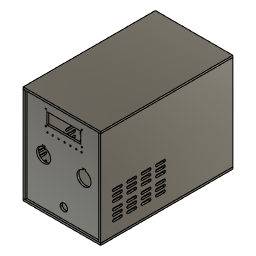
lazy-welder-chassis (Autodesk Fusion 360 design; units mm, degrees)
Autodesk Fusion 360 part; units mm, degrees
sketch "Sketch1" plane through (0, 0, 0) normal (0, 1, 0) x (1, 0, 0)
  line L0 (0, 0) -> (0, -197.9)
  line L1 (0, -197.9) -> (153.8, -197.9)
  line L2 (153.8, -197.9) -> (153.8, 0)
  line L3 (153.8, 0) -> (0, 0)
  line L4 (41.45, -177.9) -> (112.35, -177.9)
  line L5 (112.35, -177.9) -> (112.35, -153.9)
  line L6 (112.35, -153.9) -> (41.45, -153.9)
  line L7 (41.45, -153.9) -> (41.45, -177.9)
  circle A0 centre (39.4, -181.4) radius 1.5
  circle A1 centre (102.95, -140.7) radius 1.5
  circle A2 centre (113.95, -140.7) radius 1.5
  circle A3 centre (90.65, -140.7) radius 1.5
  circle A4 centre (78.35, -140.7) radius 1.5
  circle A5 centre (66.05, -140.7) radius 1.5
  circle A6 centre (53.75, -140.7) radius 1.5
  circle A7 centre (42.75, -140.7) radius 1.5
  circle A8 centre (114.4, -181.4) radius 1.5
  line L8 (31.8, -113.1111) -> (37.6, -113.1111)
  line L9 (31.8, -113.1111) -> (31.8, -110.1111)
  line L10 (37.6, -113.1111) -> (37.6, -110.1111)
  arc A9 (37.6, -110.1111) -> (31.8, -110.1111) centre (34.7, -95.7) ccw
  line L11 (116.2, -113.1111) -> (122, -113.1111)
  line L12 (116.2, -113.1111) -> (116.2, -110.1111)
  line L13 (122, -113.1111) -> (122, -110.1111)
  arc A10 (122, -110.1111) -> (116.2, -110.1111) centre (119.1, -95.7) ccw
  circle A11 centre (114.4, -150.4) radius 1.5
  circle A12 centre (39.4, -150.4) radius 1.5
  line L14 (69.55, -25.0076) -> (69.55, -20.0924)
  line L15 (84.25, -25.0076) -> (84.25, -20.0924)
  arc A13 (69.55, -25.0076) -> (84.25, -25.0076) centre (76.9, -22.55) ccw
  arc A14 (84.25, -20.0924) -> (69.55, -20.0924) centre (76.9, -22.55) ccw
  point P0 (106.0012, -102.3717)
  point P1 (41.7115, -182.3254)
  dimension "d1" = 197.9
  dimension "d6" = 70.9
  dimension "d13" = 153.8
  dimension "d22" = 29.4
  dimension "d27" = 95.7
  dimension "d28" = 34.7
  dimension "d29" = 84.4
  dimension "d30" = 95.7
  dimension "d31" = 34.7
  dimension "d32" = 22.55
  dimension "d33" = 76.9
  dimension "d34" = 20
  dimension "d35" = 41.45
  dimension "d38" = 3
  dimension "d39" = 13.2
  dimension "d40" = 9.4
  dimension "d41" = 3
  dimension "d42" = 11
  dimension "d43" = 13.2
  dimension "d44" = 3
  dimension "d45" = 3
  dimension "d46" = 12.3
  dimension "d47" = 12.3
  dimension "d49" = 12.3
  dimension "d50" = 3
  dimension "d51" = 12.3
  dimension "d52" = 3
  dimension "d53" = 11
  dimension "d54" = 13.2
  dimension "d55" = 13.2
  dimension "d56" = 13.2
  dimension "d57" = 13.2
  dimension "d58" = 3
  dimension "d59" = 13.2
  dimension "d60" = 3
  dimension "d61" = 75
  dimension "d69" = 5.8
  dimension "d70" = 3
  dimension "d71" = 3
  dimension "d72" = 5.8
  dimension "d73" = 3
  dimension "d74" = 3
  dimension "d77" = 3
  dimension "d78" = 3
  dimension "d80" = 31
  dimension "d81" = 31
  dimension "d82" = 24
  dimension "d83" = 3.5
  dimension "d86" = 75
  dimension "d87" = 2.05
  dimension "d89" = 3
  dimension "d94" = 14.7
  dimension "d101" = 14.7
  dimension "d102" = 7.75
  constraint coincident L0.start L3.end
  constraint vertical L0
  constraint perpendicular L0 L1
  constraint perpendicular L1 L2
  constraint perpendicular L0 L3
  constraint horizontal L4
  constraint vertical L5
  constraint horizontal L6
  constraint vertical L7
  constraint coincident P0 A10
  constraint horizontal L8
  constraint perpendicular L8 L9
  constraint perpendicular L8 L10
  constraint horizontal L11
  constraint perpendicular L11 L12
  constraint perpendicular L11 L13
  constraint vertical L14
  constraint coincident L15.end A13
  constraint vertical L15
  constraint concentric A13 A14
  measures "d1" distance of L0.start L0.end
  measures "d6" distance of L4.start L4.end
  measures "d13" distance of L0.end L1.end
  measures "d22" diameter of A9
  measures "d27" distance of L3 A9.centre
  measures "d28" distance of L0 A9.centre
  measures "d29" horizontal distance of A10.centre A9.centre
  measures "d30" distance of L3 A10.centre
  measures "d31" distance of L2 A10.centre
  measures "d32" distance of L3 A13.centre
  measures "d33" distance of L0 A13.centre
  measures "d34" distance of L1 L4
  measures "d35" distance of L0 L7
  measures "d38" diameter of A1
  measures "d39" distance of L6 A1.centre
  measures "d40" distance of L5 A1.centre
  measures "d41" diameter of A2
  measures "d42" horizontal distance of A1.centre A2.centre
  measures "d43" distance of L6 A2.centre
  measures "d44" diameter of A3
  measures "d45" diameter of A4
  measures "d46" horizontal distance of A1.centre A3.centre
  measures "d47" horizontal distance of A3.centre A4.centre
  measures "d49" horizontal distance of A4.centre A5.centre
  measures "d50" diameter of A6
  measures "d51" horizontal distance of A5.centre A6.centre
  measures "d52" diameter of A7
  measures "d53" distance of A6.centre A7.centre
  measures "d54" distance of L6 A3.centre
  measures "d55" distance of L6 A4.centre
  measures "d56" distance of L6 A5.centre
  measures "d57" distance of L6 A6.centre
  measures "d58" diameter of A5
  measures "d59" distance of L6 A7.centre
  measures "d60" diameter of A8
  measures "d61" horizontal distance of A0.centre A8.centre
  measures "d69" distance of L8.start L8.end
  measures "d70" distance of L8.start L9.end
  measures "d71" distance of L8.end L10.end
  measures "d72" distance of L11.start L11.end
  measures "d73" distance of L11.start L12.end
  measures "d74" distance of L11.end L13.end
  measures "d77" diameter of A11
  measures "d78" diameter of A12
  measures "d80" vertical distance of A8.centre A11.centre
  measures "d81" vertical distance of A0.centre A12.centre
  measures "d82" distance of L4.start L6.end
  measures "d83" distance of L4 A0.centre
  measures "d86" distance of A11.centre A12.centre
  measures "d87" distance of L7 A0.centre
  measures "d89" diameter of A0
  measures "d94" radius of A10
  measures "d101" distance of L14 L15
  measures "d102" radius of A13
sketch "Sketch3" plane through (0, 0, 0) normal (0, 1, 0) x (1, 0, 0)
  line L0 (0, -197.9) -> (153.8, -197.9)
  line L1 (153.8, -197.9) -> (153.8, 0)
  line L2 (153.8, 0) -> (0, 0)
  circle A0 centre (99.4, -30) radius 1.7
  circle A1 centre (139.4, -30) radius 1.7
  line L3 (112.4711, -40) -> (126.3289, -40)
  line L4 (133.4, -32.9289) -> (133.4, -24)
  line L5 (129.4, -20) -> (109.4, -20)
  line L6 (105.4, -24) -> (105.4, -32.9289)
  line L7 (105.4, -32.9289) -> (112.4711, -40)
  line L8 (105.4, -32.9289) -> (47.9841, -32.9289) construction
  line L9 (126.3289, -40) -> (133.4, -32.9289)
  line L10 (126.3289, -40) -> (50.3873, -40) construction
  arc A2 (133.4, -24) -> (129.4, -20) centre (129.4, -24) ccw
  arc A3 (109.4, -20) -> (105.4, -24) centre (109.4, -24) ccw
  line L11 (105, -71.5) -> (133.8, -71.5)
  line L12 (133.8, -71.5) -> (133.8, -50)
  line L13 (133.8, -50) -> (105, -50)
  line L14 (105, -50) -> (105, -71.5)
  circle A4 centre (22.5, -175.4037) radius 2.15
  circle A5 centre (22.5, -143.4037) radius 2.15
  circle A6 centre (54.5073, -143.4037) radius 2.15
  circle A7 centre (54.5, -175.4037) radius 2.15
  circle A8 centre (99.3, -175.4037) radius 2.15
  circle A9 centre (99.3, -143.4037) radius 2.15
  circle A10 centre (131.3, -175.4037) radius 2.15
  circle A11 centre (131.3, -143.4037) radius 2.15
  circle A12 centre (38.5, -159.4) radius 18.5
  circle A13 centre (115.3, -159.4) radius 18.5
  line L15 (0, -20) -> (17.5, -20)
  line L16 (17.5, -20) -> (17.5, -100)
  line L17 (17.5, -100) -> (0, -100)
  line L18 (0, 0) -> (0, -20)
  line L19 (0, -100) -> (0, -197.9)
  dimension "d103" = 197.9
  dimension "d104" = 153.8
  dimension "d105" = 3.4
  dimension "d106" = 3.4
  dimension "d109" = 4
  dimension "d110" = 4
  dimension "d117" = 10
  dimension "d121" = 10
  dimension "d124" = 6
  dimension "d125" = 6
  dimension "d126" = 40
  dimension "d127" = 10
  dimension "d128" = 10
  dimension "d129" = 28.8
  dimension "d130" = 21.5
  dimension "d131" = 20
  dimension "d133" = 20
  dimension "d134" = 20
  dimension "d135" = 50
  dimension "d136" = 4.3
  dimension "d137" = 4.3
  dimension "d138" = 4.3
  dimension "d139" = 4.3
  dimension "d140" = 4.3
  dimension "d141" = 4.3
  dimension "d142" = 4.3
  dimension "d143" = 4.3
  dimension "d144" = 32
  dimension "d145" = 32
  dimension "d148" = 32
  dimension "d149" = 32
  dimension "d150" = 32
  dimension "d151" = 37
  dimension "d152" = 22.63
  dimension "d153" = 22.63
  dimension "d154" = 22.63
  dimension "d155" = 22.6248
  dimension "d156" = 38.5
  dimension "d157" = 38.5
  dimension "d158" = 32
  dimension "d159" = 32
  dimension "d160" = 32
  dimension "d161" = 32
  dimension "d162" = 32
  dimension "d163" = 32
  dimension "d164" = 37
  dimension "d165" = 22.63
  dimension "d166" = 22.63
  dimension "d167" = 22.6248
  dimension "d168" = 22.6248
  dimension "d169" = 38.5
  dimension "d170" = 38.5
  dimension "d310" = 20.4
  dimension "d311" = 17.5
  dimension "d312" = 80
  dimension "d313" = 20
  constraint coincident L2.end L18.start
  constraint vertical L18
  constraint perpendicular L0 L18
  constraint perpendicular L0 L1
  constraint perpendicular L2 L18
  constraint horizontal L3
  constraint vertical L4
  constraint horizontal L5
  constraint vertical L6
  constraint tangent L6 A3
  constraint tangent L5 A3
  constraint tangent L4 A2
  constraint tangent L5 A2
  constraint horizontal L8
  constraint horizontal L10
  constraint horizontal L11
  constraint vertical L12
  constraint horizontal L13
  constraint vertical L14
  constraint perpendicular L15 L18
  constraint perpendicular L15 L16
  constraint coincident L17.end L18
  constraint perpendicular L17 L18
  constraint collinear L18 L19
  measures "d103" distance of L2.end L0.start
  measures "d104" distance of L0.start L0.end
  measures "d105" diameter of A0
  measures "d106" diameter of A1
  measures "d109" radius of A3
  measures "d110" radius of A2
  measures "d117" distance of A0.centre L3
  measures "d121" distance of A1.centre L3
  measures "d124" distance of A0.centre L6
  measures "d125" distance of A1.centre L4
  measures "d126" distance of A0.centre A1.centre
  measures "d127" distance of L6.end L3.start
  measures "d128" distance of L3.end L4.start
  measures "d129" distance of L11.start L11.end
  measures "d130" distance of L11.start L13.end
  measures "d131" distance of L3 L5
  measures "d133" distance of L2 L5
  measures "d134" distance of L1 L12
  measures "d135" distance of L2 L13
  measures "d136" diameter of A4
  measures "d137" diameter of A5
  measures "d138" diameter of A6
  measures "d139" diameter of A7
  measures "d140" diameter of A8
  measures "d141" diameter of A9
  measures "d142" diameter of A10
  measures "d143" diameter of A11
  measures "d144" horizontal distance of A4.centre A7.centre
  measures "d145" vertical distance of A4.centre A5.centre
  measures "d148" vertical distance of A5.centre A7.centre
  measures "d149" horizontal distance of A5.centre A7.centre
  measures "d150" distance of A6.centre A7.centre
  measures "d151" diameter of A12
  measures "d152" distance of A4.centre A12.centre
  measures "d153" distance of A7.centre A12.centre
  measures "d154" distance of A6.centre A12.centre
  measures "d155" distance of A5.centre A12.centre
  measures "d156" distance of L0 A12.centre
  measures "d157" distance of A12.centre L18
  measures "d158" horizontal distance of A8.centre A10.centre
  measures "d159" horizontal distance of A9.centre A10.centre
  measures "d160" horizontal distance of A8.centre A11.centre
  measures "d161" distance of A8.centre A9.centre
  measures "d162" vertical distance of A8.centre A11.centre
  measures "d163" distance of A10.centre A11.centre
  measures "d164" diameter of A13
  measures "d165" distance of A8.centre A13.centre
  measures "d166" distance of A10.centre A13.centre
  measures "d167" distance of A9.centre A13.centre
  measures "d168" distance of A11.centre A13.centre
  measures "d169" distance of L0 A13.centre
  measures "d170" distance of L1 A13.centre
  measures "d310" distance of L1 L4
  measures "d311" distance of L15.start L15.end
  measures "d312" distance of L15.end L16.end
  measures "d313" distance of L2 L15
extrude "Extrude3" add sketch "Sketch1" along normal blind 4 makes body 1
extrude "Extrude4" add sketch "Sketch3" along normal blind 4 separate body makes body 2
move_face "MoveFace1" by (0, 0, 260) 1 faces at (153.8, 1.3333, 131.9333) on bodies 2
move_body "Move1" bodies 2 to x (1, 0, 0) y (0, 1, 0) z (0, 0, 1) at (0, 263, 0)
sketch "Sketch4" plane through (0, 0, 0) normal (1, 0, 0) x (0, 1, 0)
  line L0 (0, 0) -> (0, 197.9)
  line L1 (0, 197.9) -> (276, 197.9)
  line L2 (276, 197.9) -> (276, 0)
  line L3 (276, 0) -> (0, 0)
  line L4 (27, 30) -> (43, 30)
  line L5 (45, 28) -> (45, 27)
  line L6 (43, 25) -> (27, 25)
  line L7 (25, 27) -> (25, 28)
  arc A0 (27, 30) -> (25, 28) centre (27, 28) ccw
  arc A1 (25, 27) -> (27, 25) centre (27, 27) ccw
  arc A2 (45, 28) -> (43, 30) centre (43, 28) ccw
  arc A3 (43, 25) -> (45, 27) centre (43, 27) ccw
  arc A4 (45, 38) -> (43, 40) centre (43, 38) ccw
  line L8 (43, 35) -> (27, 35)
  arc A5 (43, 35) -> (45, 37) centre (43, 37) ccw
  line L9 (27, 40) -> (43, 40)
  line L10 (45, 38) -> (45, 37)
  arc A6 (27, 40) -> (25, 38) centre (27, 38) ccw
  arc A7 (25, 37) -> (27, 35) centre (27, 37) ccw
  line L11 (25, 37) -> (25, 38)
  arc A8 (45, 48) -> (43, 50) centre (43, 48) ccw
  line L12 (43, 45) -> (27, 45)
  arc A9 (43, 45) -> (45, 47) centre (43, 47) ccw
  line L13 (27, 50) -> (43, 50)
  line L14 (45, 48) -> (45, 47)
  arc A10 (27, 50) -> (25, 48) centre (27, 48) ccw
  arc A11 (25, 47) -> (27, 45) centre (27, 47) ccw
  line L15 (25, 47) -> (25, 48)
  arc A12 (75, 28) -> (73, 30) centre (73, 28) ccw
  line L16 (73, 25) -> (57, 25)
  arc A13 (73, 25) -> (75, 27) centre (73, 27) ccw
  line L17 (57, 30) -> (73, 30)
  line L18 (75, 28) -> (75, 27)
  arc A14 (57, 30) -> (55, 28) centre (57, 28) ccw
  arc A15 (55, 27) -> (57, 25) centre (57, 27) ccw
  line L19 (55, 27) -> (55, 28)
  arc A16 (75, 38) -> (73, 40) centre (73, 38) ccw
  line L20 (73, 35) -> (57, 35)
  arc A17 (73, 35) -> (75, 37) centre (73, 37) ccw
  line L21 (57, 40) -> (73, 40)
  line L22 (75, 38) -> (75, 37)
  arc A18 (57, 40) -> (55, 38) centre (57, 38) ccw
  arc A19 (55, 37) -> (57, 35) centre (57, 37) ccw
  line L23 (55, 37) -> (55, 38)
  arc A20 (75, 48) -> (73, 50) centre (73, 48) ccw
  line L24 (73, 45) -> (57, 45)
  arc A21 (73, 45) -> (75, 47) centre (73, 47) ccw
  line L25 (57, 50) -> (73, 50)
  line L26 (75, 48) -> (75, 47)
  arc A22 (57, 50) -> (55, 48) centre (57, 48) ccw
  arc A23 (55, 47) -> (57, 45) centre (57, 47) ccw
  line L27 (55, 47) -> (55, 48)
  arc A24 (105, 28) -> (103, 30) centre (103, 28) ccw
  line L28 (103, 25) -> (87, 25)
  arc A25 (103, 25) -> (105, 27) centre (103, 27) ccw
  line L29 (87, 30) -> (103, 30)
  line L30 (105, 28) -> (105, 27)
  arc A26 (87, 30) -> (85, 28) centre (87, 28) ccw
  arc A27 (85, 27) -> (87, 25) centre (87, 27) ccw
  line L31 (85, 27) -> (85, 28)
  arc A28 (105, 38) -> (103, 40) centre (103, 38) ccw
  line L32 (103, 35) -> (87, 35)
  arc A29 (103, 35) -> (105, 37) centre (103, 37) ccw
  line L33 (87, 40) -> (103, 40)
  line L34 (105, 38) -> (105, 37)
  arc A30 (87, 40) -> (85, 38) centre (87, 38) ccw
  arc A31 (85, 37) -> (87, 35) centre (87, 37) ccw
  line L35 (85, 37) -> (85, 38)
  arc A32 (105, 48) -> (103, 50) centre (103, 48) ccw
  line L36 (103, 45) -> (87, 45)
  arc A33 (103, 45) -> (105, 47) centre (103, 47) ccw
  line L37 (87, 50) -> (103, 50)
  line L38 (105, 48) -> (105, 47)
  arc A34 (87, 50) -> (85, 48) centre (87, 48) ccw
  arc A35 (85, 47) -> (87, 45) centre (87, 47) ccw
  line L39 (85, 47) -> (85, 48)
  arc A36 (135, 28) -> (133, 30) centre (133, 28) ccw
  line L40 (133, 25) -> (117, 25)
  arc A37 (133, 25) -> (135, 27) centre (133, 27) ccw
  line L41 (117, 30) -> (133, 30)
  line L42 (135, 28) -> (135, 27)
  arc A38 (117, 30) -> (115, 28) centre (117, 28) ccw
  arc A39 (115, 27) -> (117, 25) centre (117, 27) ccw
  line L43 (115, 27) -> (115, 28)
  arc A40 (135, 38) -> (133, 40) centre (133, 38) ccw
  line L44 (133, 35) -> (117, 35)
  arc A41 (133, 35) -> (135, 37) centre (133, 37) ccw
  line L45 (117, 40) -> (133, 40)
  line L46 (135, 38) -> (135, 37)
  arc A42 (117, 40) -> (115, 38) centre (117, 38) ccw
  arc A43 (115, 37) -> (117, 35) centre (117, 37) ccw
  line L47 (115, 37) -> (115, 38)
  arc A44 (135, 48) -> (133, 50) centre (133, 48) ccw
  line L48 (133, 45) -> (117, 45)
  arc A45 (133, 45) -> (135, 47) centre (133, 47) ccw
  line L49 (117, 50) -> (133, 50)
  line L50 (135, 48) -> (135, 47)
  arc A46 (117, 50) -> (115, 48) centre (117, 48) ccw
  arc A47 (115, 47) -> (117, 45) centre (117, 47) ccw
  line L51 (115, 47) -> (115, 48)
  arc A48 (45, 28) -> (43, 30) centre (43, 28) ccw
  line L52 (43, 25) -> (27, 25)
  arc A49 (43, 25) -> (45, 27) centre (43, 27) ccw
  line L53 (27, 30) -> (43, 30)
  line L54 (45, 28) -> (45, 27)
  arc A50 (27, 30) -> (25, 28) centre (27, 28) ccw
  arc A51 (25, 27) -> (27, 25) centre (27, 27) ccw
  line L55 (25, 27) -> (25, 28)
  line L56 (57, 65) -> (73, 65)
  arc A52 (85, 72) -> (87, 70) centre (87, 72) ccw
  line L57 (85, 62) -> (85, 63)
  arc A53 (73, 70) -> (75, 72) centre (73, 72) ccw
  arc A54 (133, 70) -> (135, 72) centre (133, 72) ccw
  arc A55 (87, 65) -> (85, 63) centre (87, 63) ccw
  arc A56 (115, 72) -> (117, 70) centre (117, 72) ccw
  line L58 (133, 70) -> (117, 70)
  line L59 (55, 82) -> (55, 83)
  arc A57 (105, 73) -> (103, 75) centre (103, 73) ccw
  line L60 (105, 63) -> (105, 62)
  line L61 (75, 83) -> (75, 82)
  arc A58 (55, 72) -> (57, 70) centre (57, 72) ccw
  line L62 (45, 73) -> (45, 72)
  arc A59 (43, 80) -> (45, 82) centre (43, 82) ccw
  arc A60 (85, 62) -> (87, 60) centre (87, 62) ccw
  line L63 (103, 70) -> (87, 70)
  line L64 (45, 63) -> (45, 62)
  line L65 (85, 82) -> (85, 83)
  arc A61 (75, 73) -> (73, 75) centre (73, 73) ccw
  line L66 (45, 63) -> (45, 62)
  line L67 (57, 85) -> (73, 85)
  arc A62 (87, 85) -> (85, 83) centre (87, 83) ccw
  line L68 (73, 60) -> (57, 60)
  line L69 (105, 73) -> (105, 72)
  line L70 (57, 75) -> (73, 75)
  arc A63 (43, 70) -> (45, 72) centre (43, 72) ccw
  line L71 (135, 83) -> (135, 82)
  arc A64 (45, 73) -> (43, 75) centre (43, 73) ccw
  arc A65 (133, 60) -> (135, 62) centre (133, 62) ccw
  arc A66 (55, 82) -> (57, 80) centre (57, 82) ccw
  arc A67 (105, 63) -> (103, 65) centre (103, 63) ccw
  arc A68 (55, 62) -> (57, 60) centre (57, 62) ccw
  line L72 (105, 83) -> (105, 82)
  line L73 (87, 85) -> (103, 85)
  arc A69 (105, 83) -> (103, 85) centre (103, 83) ccw
  line L74 (103, 80) -> (87, 80)
  arc A70 (85, 82) -> (87, 80) centre (87, 82) ccw
  line L75 (43, 60) -> (27, 60)
  line L76 (27, 65) -> (43, 65)
  arc A71 (25, 62) -> (27, 60) centre (27, 62) ccw
  arc A72 (27, 75) -> (25, 73) centre (27, 73) ccw
  line L77 (73, 70) -> (57, 70)
  line L78 (73, 80) -> (57, 80)
  arc A73 (45, 63) -> (43, 65) centre (43, 63) ccw
  arc A74 (45, 83) -> (43, 85) centre (43, 83) ccw
  line L79 (55, 62) -> (55, 63)
  arc A75 (43, 60) -> (45, 62) centre (43, 62) ccw
  line L80 (117, 85) -> (133, 85)
  line L81 (115, 72) -> (115, 73)
  line L82 (135, 73) -> (135, 72)
  line L83 (87, 75) -> (103, 75)
  arc A76 (57, 75) -> (55, 73) centre (57, 73) ccw
  line L84 (85, 72) -> (85, 73)
  arc A77 (103, 70) -> (105, 72) centre (103, 72) ccw
  arc A78 (135, 63) -> (133, 65) centre (133, 63) ccw
  arc A79 (73, 60) -> (75, 62) centre (73, 62) ccw
  arc A80 (43, 60) -> (45, 62) centre (43, 62) ccw
  arc A81 (57, 65) -> (55, 63) centre (57, 63) ccw
  line L85 (75, 73) -> (75, 72)
  arc A82 (87, 75) -> (85, 73) centre (87, 73) ccw
  arc A83 (103, 60) -> (105, 62) centre (103, 62) ccw
  line L86 (55, 72) -> (55, 73)
  line L87 (87, 65) -> (103, 65)
  arc A84 (135, 73) -> (133, 75) centre (133, 73) ccw
  line L88 (117, 65) -> (133, 65)
  arc A85 (45, 63) -> (43, 65) centre (43, 63) ccw
  arc A86 (75, 63) -> (73, 65) centre (73, 63) ccw
  arc A87 (115, 82) -> (117, 80) centre (117, 82) ccw
  arc A88 (75, 83) -> (73, 85) centre (73, 83) ccw
  arc A89 (133, 80) -> (135, 82) centre (133, 82) ccw
  arc A90 (57, 85) -> (55, 83) centre (57, 83) ccw
  line L89 (27, 85) -> (43, 85)
  line L90 (25, 62) -> (25, 63)
  line L91 (27, 75) -> (43, 75)
  line L92 (117, 75) -> (133, 75)
  line L93 (25, 82) -> (25, 83)
  arc A91 (115, 62) -> (117, 60) centre (117, 62) ccw
  line L94 (43, 60) -> (27, 60)
  arc A92 (25, 82) -> (27, 80) centre (27, 82) ccw
  arc A93 (117, 65) -> (115, 63) centre (117, 63) ccw
  line L95 (45, 83) -> (45, 82)
  arc A94 (73, 80) -> (75, 82) centre (73, 82) ccw
  arc A95 (25, 72) -> (27, 70) centre (27, 72) ccw
  line L96 (43, 80) -> (27, 80)
  arc A96 (25, 62) -> (27, 60) centre (27, 62) ccw
  line L97 (115, 82) -> (115, 83)
  line L98 (43, 70) -> (27, 70)
  arc A97 (117, 75) -> (115, 73) centre (117, 73) ccw
  line L99 (135, 63) -> (135, 62)
  arc A98 (117, 85) -> (115, 83) centre (117, 83) ccw
  line L100 (103, 60) -> (87, 60)
  arc A99 (103, 80) -> (105, 82) centre (103, 82) ccw
  arc A100 (27, 65) -> (25, 63) centre (27, 63) ccw
  arc A101 (27, 65) -> (25, 63) centre (27, 63) ccw
  line L101 (27, 65) -> (43, 65)
  line L102 (25, 62) -> (25, 63)
  line L103 (133, 60) -> (117, 60)
  line L104 (133, 80) -> (117, 80)
  line L105 (115, 62) -> (115, 63)
  arc A102 (135, 83) -> (133, 85) centre (133, 83) ccw
  line L106 (25, 72) -> (25, 73)
  line L107 (75, 63) -> (75, 62)
  arc A103 (27, 85) -> (25, 83) centre (27, 83) ccw
  dimension "d178" = 197.9
  dimension "d179" = 276
  dimension "d190" = 2
  dimension "d191" = 2
  dimension "d192" = 2
  dimension "d193" = 2
  dimension "d194" = 2
  dimension "d195" = 2
  dimension "d196" = 2
  dimension "d197" = 2
  dimension "d198" = 2
  dimension "d199" = 2
  dimension "d200" = 2
  dimension "d201" = 2
  dimension "d202" = 2
  dimension "d203" = 2
  dimension "d204" = 2
  dimension "d205" = 2
  dimension "d206" = 2
  dimension "d207" = 2
  dimension "d208" = 2
  dimension "d209" = 2
  dimension "d210" = 2
  dimension "d211" = 2
  dimension "d212" = 2
  dimension "d213" = 2
  dimension "d214" = 2
  dimension "d215" = 2
  dimension "d216" = 2
  dimension "d217" = 2
  dimension "d218" = 2
  dimension "d219" = 2
  dimension "d220" = 2
  dimension "d221" = 2
  dimension "d222" = 2
  dimension "d223" = 2
  dimension "d224" = 2
  dimension "d225" = 2
  dimension "d226" = 2
  dimension "d227" = 2
  dimension "d228" = 2
  dimension "d229" = 2
  dimension "d230" = 2
  dimension "d231" = 2
  dimension "d232" = 2
  dimension "d233" = 2
  dimension "d234" = 2
  dimension "d235" = 2
  dimension "d236" = 2
  dimension "d237" = 2
  dimension "d238" = 2
  dimension "d239" = 2
  dimension "d240" = 2
  dimension "d241" = 2
  dimension "d242" = 2
  dimension "d243" = 2
  dimension "d244" = 2
  dimension "d245" = 2
  dimension "d246" = 2
  dimension "d247" = 2
  dimension "d248" = 2
  dimension "d249" = 2
  dimension "d250" = 2
  dimension "d251" = 2
  dimension "d252" = 2
  dimension "d253" = 2
  dimension "d254" = 2
  dimension "d255" = 2
  dimension "d256" = 2
  dimension "d257" = 2
  dimension "d258" = 2
  dimension "d259" = 2
  dimension "d260" = 2
  dimension "d261" = 2
  dimension "d262" = 2
  dimension "d263" = 2
  dimension "d264" = 2
  dimension "d265" = 2
  dimension "d266" = 2
  dimension "d267" = 2
  dimension "d268" = 2
  dimension "d269" = 2
  dimension "d270" = 2
  dimension "d271" = 2
  dimension "d272" = 2
  dimension "d273" = 2
  dimension "d274" = 2
  dimension "d275" = 2
  dimension "d276" = 2
  dimension "d277" = 2
  dimension "d278" = 2
  dimension "d279" = 2
  dimension "d280" = 2
  dimension "d281" = 2
  dimension "d282" = 2
  dimension "d283" = 2
  dimension "d284" = 2
  dimension "d285" = 2
  dimension "d286" = 2
  dimension "d287" = 2
  dimension "d288" = 2
  dimension "d289" = 2
  dimension "d290" = 2
  dimension "d291" = 2
  dimension "d292" = 2
  dimension "d293" = 2
  constraint coincident L0.start L3.end
  constraint vertical L0
  constraint perpendicular L0 L1
  constraint perpendicular L1 L2
  constraint perpendicular L0 L3
  constraint horizontal L4
  constraint vertical L5
  constraint horizontal L6
  constraint vertical L7
  constraint tangent L4 A0
  constraint tangent L7 A0
  constraint tangent L6 A1
  constraint tangent L7 A1
  constraint tangent L4 A2
  constraint tangent L5 A2
  constraint tangent L5 A3
  constraint tangent L6 A3
  constraint horizontal L9
  constraint vertical L10
  constraint horizontal L8
  constraint vertical L11
  constraint tangent L9 A6
  constraint tangent A6 L11
  constraint tangent L8 A7
  constraint tangent A7 L11
  constraint tangent A4 L9
  constraint tangent A4 L10
  constraint tangent A5 L10
  constraint tangent L8 A5
  constraint horizontal L13
  constraint vertical L14
  constraint horizontal L12
  constraint vertical L15
  constraint tangent L13 A10
  constraint tangent A10 L15
  constraint tangent L12 A11
  constraint tangent A11 L15
  constraint tangent A8 L13
  constraint tangent A8 L14
  constraint tangent A9 L14
  constraint tangent L12 A9
  constraint horizontal L17
  constraint vertical L18
  constraint horizontal L16
  constraint vertical L19
  constraint tangent L17 A14
  constraint tangent A14 L19
  constraint tangent L16 A15
  constraint tangent A15 L19
  constraint tangent A12 L17
  constraint tangent A12 L18
  constraint tangent A13 L18
  constraint tangent L16 A13
  constraint horizontal L21
  constraint vertical L22
  constraint horizontal L20
  constraint vertical L23
  constraint tangent L21 A18
  constraint tangent A18 L23
  constraint tangent L20 A19
  constraint tangent A19 L23
  constraint tangent A16 L21
  constraint tangent A16 L22
  constraint tangent A17 L22
  constraint tangent L20 A17
  constraint horizontal L25
  constraint vertical L26
  constraint horizontal L24
  constraint vertical L27
  constraint tangent L25 A22
  constraint tangent A22 L27
  constraint tangent L24 A23
  constraint tangent A23 L27
  constraint tangent A20 L25
  constraint tangent A20 L26
  constraint tangent A21 L26
  constraint tangent L24 A21
  constraint horizontal L29
  constraint vertical L30
  constraint horizontal L28
  constraint vertical L31
  constraint tangent L29 A26
  constraint tangent A26 L31
  constraint tangent L28 A27
  constraint tangent A27 L31
  constraint tangent A24 L29
  constraint tangent A24 L30
  constraint tangent A25 L30
  constraint tangent L28 A25
  constraint horizontal L33
  constraint vertical L34
  constraint horizontal L32
  constraint vertical L35
  constraint tangent L33 A30
  constraint tangent A30 L35
  constraint tangent L32 A31
  constraint tangent A31 L35
  constraint tangent A28 L33
  constraint tangent A28 L34
  constraint tangent A29 L34
  constraint tangent L32 A29
  constraint horizontal L37
  constraint vertical L38
  constraint horizontal L36
  constraint vertical L39
  constraint tangent L37 A34
  constraint tangent A34 L39
  constraint tangent L36 A35
  constraint tangent A35 L39
  constraint tangent A32 L37
  constraint tangent A32 L38
  constraint tangent A33 L38
  constraint tangent L36 A33
  constraint horizontal L41
  constraint vertical L42
  constraint horizontal L40
  constraint vertical L43
  constraint tangent L41 A38
  constraint tangent A38 L43
  constraint tangent L40 A39
  constraint tangent A39 L43
  constraint tangent A36 L41
  constraint tangent A36 L42
  constraint tangent A37 L42
  constraint tangent L40 A37
  constraint horizontal L45
  constraint vertical L46
  constraint horizontal L44
  constraint vertical L47
  constraint tangent L45 A42
  constraint tangent A42 L47
  constraint tangent L44 A43
  constraint tangent A43 L47
  constraint tangent A40 L45
  constraint tangent A40 L46
  constraint tangent A41 L46
  constraint tangent L44 A41
  constraint horizontal L49
  constraint vertical L50
  constraint horizontal L48
  constraint vertical L51
  constraint tangent L49 A46
  constraint tangent A46 L51
  constraint tangent L48 A47
  constraint tangent A47 L51
  constraint tangent A44 L49
  constraint tangent A44 L50
  constraint tangent A45 L50
  constraint tangent L48 A45
  constraint horizontal L53
  constraint vertical L54
  constraint horizontal L52
  constraint vertical L55
  constraint tangent L53 A50
  constraint tangent A50 L55
  constraint tangent L52 A51
  constraint tangent A51 L55
  constraint tangent A48 L53
  constraint tangent A48 L54
  constraint tangent A49 L54
  constraint tangent L52 A49
  constraint horizontal L101
  constraint vertical L64
  constraint horizontal L94
  constraint vertical L90
  constraint tangent A100 L101
  constraint tangent L90 A100
  constraint tangent L94 A96
  constraint tangent L90 A96
  constraint tangent A73 L101
  constraint tangent L64 A73
  constraint tangent L64 A80
  constraint tangent A80 L94
  constraint horizontal L91
  constraint vertical L62
  constraint horizontal L98
  constraint vertical L106
  constraint tangent A72 L91
  constraint tangent A72 L106
  constraint tangent A95 L98
  constraint tangent A95 L106
  constraint tangent A64 L91
  constraint tangent L62 A64
  constraint tangent L62 A63
  constraint tangent A63 L98
  constraint horizontal L89
  constraint vertical L95
  constraint horizontal L96
  constraint vertical L93
  constraint tangent L89 A103
  constraint tangent L93 A103
  constraint tangent A92 L96
  constraint tangent L93 A92
  constraint tangent A74 L89
  constraint tangent A74 L95
  constraint tangent A59 L95
  constraint tangent A59 L96
  constraint horizontal L56
  constraint vertical L107
  constraint horizontal L68
  constraint vertical L79
  constraint tangent L56 A81
  constraint tangent L79 A81
  constraint tangent L68 A68
  constraint tangent A68 L79
  constraint tangent L56 A86
  constraint tangent A86 L107
  constraint tangent A79 L107
  constraint tangent L68 A79
  constraint horizontal L70
  constraint vertical L85
  constraint horizontal L77
  constraint vertical L86
  constraint tangent L70 A76
  constraint tangent A76 L86
  constraint tangent A58 L77
  constraint tangent A58 L86
  constraint tangent A61 L70
  constraint tangent A61 L85
  constraint tangent A53 L85
  constraint tangent A53 L77
  constraint horizontal L67
  constraint vertical L61
  constraint horizontal L78
  constraint vertical L59
  constraint tangent L67 A90
  constraint tangent L59 A90
  constraint tangent A66 L78
  constraint tangent L59 A66
  constraint tangent L67 A88
  constraint tangent L61 A88
  constraint tangent L61 A94
  constraint tangent L78 A94
  constraint horizontal L87
  constraint vertical L60
  constraint horizontal L100
  constraint vertical L57
  constraint tangent A55 L87
  constraint tangent L57 A55
  constraint tangent A60 L100
  constraint tangent L57 A60
  constraint tangent A67 L87
  constraint tangent L60 A67
  constraint tangent L60 A83
  constraint tangent A83 L100
  constraint horizontal L83
  constraint vertical L69
  constraint horizontal L63
  constraint vertical L84
  constraint tangent L83 A82
  constraint tangent L84 A82
  constraint tangent A52 L63
  constraint tangent A52 L84
  constraint tangent A57 L83
  constraint tangent A57 L69
  constraint tangent L69 A77
  constraint tangent L63 A77
  constraint horizontal L73
  constraint vertical L72
  constraint horizontal L74
  constraint vertical L65
  constraint tangent A62 L73
  constraint tangent L65 A62
  constraint tangent L74 A70
  constraint tangent L65 A70
  constraint tangent L73 A69
  constraint tangent L72 A69
  constraint tangent L72 A99
  constraint tangent L74 A99
  constraint horizontal L88
  constraint vertical L99
  constraint horizontal L103
  constraint vertical L105
  constraint tangent L88 A93
  constraint tangent A93 L105
  constraint tangent A91 L103
  constraint tangent A91 L105
  constraint tangent A78 L88
  constraint tangent A78 L99
  constraint tangent A65 L99
  constraint tangent A65 L103
  constraint horizontal L92
  constraint vertical L82
  constraint horizontal L58
  constraint vertical L81
  constraint tangent L92 A97
  constraint tangent L81 A97
  constraint tangent A56 L58
  constraint tangent A56 L81
  constraint tangent A84 L92
  constraint tangent L82 A84
  constraint tangent A54 L82
  constraint tangent A54 L58
  constraint horizontal L80
  constraint vertical L71
  constraint horizontal L104
  constraint vertical L97
  constraint tangent L80 A98
  constraint tangent L97 A98
  constraint tangent A87 L104
  constraint tangent A87 L97
  constraint tangent L80 A102
  constraint tangent L71 A102
  constraint tangent L71 A89
  constraint tangent A89 L104
  constraint horizontal L76
  constraint vertical L66
  constraint horizontal L75
  constraint vertical L102
  constraint tangent L76 A101
  constraint tangent A101 L102
  constraint tangent L75 A71
  constraint tangent A71 L102
  constraint tangent L76 A85
  constraint tangent L66 A85
  constraint tangent L66 A75
  constraint tangent L75 A75
  measures "d178" distance of L0.start L0.end
  measures "d179" distance of L0.end L1.end
  measures "d190" radius of A0
  measures "d191" radius of A1
  measures "d192" radius of A2
  measures "d193" radius of A3
  measures "d194" radius of A6
  measures "d195" radius of A7
  measures "d196" radius of A4
  measures "d197" radius of A5
  measures "d198" radius of A10
  measures "d199" radius of A11
  measures "d200" radius of A8
  measures "d201" radius of A9
  measures "d202" radius of A14
  measures "d203" radius of A15
  measures "d204" radius of A12
  measures "d205" radius of A13
  measures "d206" radius of A18
  measures "d207" radius of A19
  measures "d208" radius of A16
  measures "d209" radius of A17
  measures "d210" radius of A22
  measures "d211" radius of A23
  measures "d212" radius of A20
  measures "d213" radius of A21
  measures "d214" radius of A26
  measures "d215" radius of A27
  measures "d216" radius of A24
  measures "d217" radius of A25
  measures "d218" radius of A30
  measures "d219" radius of A31
  measures "d220" radius of A28
  measures "d221" radius of A29
  measures "d222" radius of A34
  measures "d223" radius of A35
  measures "d224" radius of A32
  measures "d225" radius of A33
  measures "d226" radius of A38
  measures "d227" radius of A39
  measures "d228" radius of A36
  measures "d229" radius of A37
  measures "d230" radius of A42
  measures "d231" radius of A43
  measures "d232" radius of A40
  measures "d233" radius of A41
  measures "d234" radius of A46
  measures "d235" radius of A47
  measures "d236" radius of A44
  measures "d237" radius of A45
  measures "d238" radius of A50
  measures "d239" radius of A51
  measures "d240" radius of A48
  measures "d241" radius of A49
  measures "d242" radius of A100
  measures "d243" radius of A96
  measures "d244" radius of A73
  measures "d245" radius of A80
  measures "d246" radius of A72
  measures "d247" radius of A95
  measures "d248" radius of A64
  measures "d249" radius of A63
  measures "d250" radius of A103
  measures "d251" radius of A92
  measures "d252" radius of A74
  measures "d253" radius of A59
  measures "d254" radius of A81
  measures "d255" radius of A68
  measures "d256" radius of A86
  measures "d257" radius of A79
  measures "d258" radius of A76
  measures "d259" radius of A58
  measures "d260" radius of A61
  measures "d261" radius of A53
  measures "d262" radius of A90
  measures "d263" radius of A66
  measures "d264" radius of A88
  measures "d265" radius of A94
  measures "d266" radius of A55
  measures "d267" radius of A60
  measures "d268" radius of A67
  measures "d269" radius of A83
  measures "d270" radius of A82
  measures "d271" radius of A52
  measures "d272" radius of A57
  measures "d273" radius of A77
  measures "d274" radius of A62
  measures "d275" radius of A70
  measures "d276" radius of A69
  measures "d277" radius of A99
  measures "d278" radius of A93
  measures "d279" radius of A91
  measures "d280" radius of A78
  measures "d281" radius of A65
  measures "d282" radius of A97
  measures "d283" radius of A56
  measures "d284" radius of A84
  measures "d285" radius of A54
  measures "d286" radius of A98
  measures "d287" radius of A87
  measures "d288" radius of A102
  measures "d289" radius of A89
  measures "d290" radius of A101
  measures "d291" radius of A71
  measures "d292" radius of A85
  measures "d293" radius of A75
move_body "Move2" bodies 2 to x (1, 0, 0) y (0, 1, 0) z (0, 0, 1) at (0, 3, 0)
move_body "Move4" bodies 1 to x (1, 0, 0) y (0, 1, 0) z (0, 0, 1) at (0, 3, 0)
sketch "Sketch6" plane through (0, 0, 0) normal (0, 0, 1) x (1, 0, 0)
  line L0 (0, 0) -> (0, 276)
  line L1 (0, 276) -> (161.8, 276)
  line L2 (161.8, 276) -> (161.8, 0)
  line L3 (161.8, 0) -> (0, 0)
  dimension "d184" = 276
  dimension "d185" = 161.8
  constraint coincident L0.start L3.end
  constraint vertical L0
  constraint perpendicular L0 L1
  constraint perpendicular L1 L2
  constraint perpendicular L0 L3
  measures "d184" distance of L0.start L0.end
  measures "d185" distance of L0.end L1.end
move_body "Move6" bodies 1 to x (1, 0, 0) y (0, 1, 0) z (0, 0, 1) at (0, 0, 3)
move_body "Move7" bodies 2 to x (1, 0, 0) y (0, 1, 0) z (0, 0, 1) at (0, 0, 3)
move_body "Move12" bodies 2 to x (1, 0, 0) y (0, 1, 0) z (0, 0, 1) at (3, 0, 0)
move_body "Move13" bodies 1 to x (1, 0, 0) y (0, 1, 0) z (0, 0, 1) at (3, 0, 0)
move_body "Move17" bodies 2 to x (1, 0, 0) y (0, 1, 0) z (0, 0, 1) at (0, -1, 0)
sketch "Sketch7" plane through (0, 0, 0) normal (0, 0, 1) x (1, 0, 0)
  line L0 (0, 0) -> (0, 260)
  line L1 (0, 260) -> (153.8, 260)
  line L2 (153.8, 260) -> (153.8, 0)
  line L3 (153.8, 0) -> (0, 0)
  dimension "d298" = 260
  dimension "d299" = 153.8
  constraint coincident L0.start L3.end
  constraint vertical L0
  constraint perpendicular L0 L1
  constraint perpendicular L1 L2
  constraint perpendicular L0 L3
  measures "d298" distance of L0.start L0.end
  measures "d299" distance of L0.end L1.end
extrude "Extrude11" add sketch "Sketch7" along normal blind 4 separate body makes body 3
move_body "Move18" bodies 3 to x (1, 0, 0) y (0, 1, 0) z (0, 0, 1) at (0, 0, 4)
move_body "Move19" bodies 3 to x (1, 0, 0) y (0, 1, 0) z (0, 0, 1) at (4, 0, 0)
move_body "Move20" bodies 2 to x (1, 0, 0) y (0, 1, 0) z (0, 0, 1) at (1, 0, 0)
move_body "Move21" bodies 1 to x (1, 0, 0) y (0, 1, 0) z (0, 0, 1) at (1, 0, 0)
move_body "Move22" bodies 1 to x (1, 0, 0) y (0, 1, 0) z (0, 0, 1) at (0, 1, 1)
move_body "Move23" bodies 3 to x (1, 0, 0) y (0, 1, 0) z (0, 0, 1) at (0, 8, 0)
move_body "Move24" bodies 2 to x (1, 0, 0) y (0, 1, 0) z (0, 0, 1) at (0, 3, 1)
extrude "Extrude12" add sketch "Sketch4" along normal blind 4 separate body makes body 4
move_body "Move25" bodies 4 to x (1, 0, 0) y (0, 1, 0) z (0, 0, 1) at (0, 0, 4)
extrude "Extrude13" add sketch "Sketch4" along normal blind 4 separate body makes body 5
move_body "Move26" bodies 5 to x (1, 0, 0) y (0, 1, 0) z (0, 0, 1) at (157.8, 0, 4)
extrude "Extrude14" add sketch "Sketch6" along normal blind 4 separate body makes body 6
extrude "Extrude15" add sketch "Sketch6" along normal blind 4 separate body makes body 7
move_body "Move27" bodies 7 to x (1, 0, 0) y (0, 1, 0) z (0, 0, 1) at (0, 0, 201.9)
